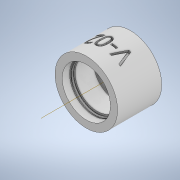
# Autodesk Inventor part: brakeStopAndOuterHousing
Saved by Autodesk Inventor 2021.1 (Build 251245000, 245)
## iProperties
Created: 2020-08-18
Part Number: brakeStopAndOuterHousing
Material: Generic
Document SubType Name: Modeling
Designer: robst
Density: 1 g/cm^3
Appearance: Default
Author: robst
Autodesk Inventor part; units mm, degrees
ref_plane "YZ Plane" through (0, 0, 0) normal (1, 0, 0) x (0, 1, 0)
ref_plane "XY Plane" through (0, 0, 0) normal (0, 0, 1) x (1, 0, 0)
sketch "Sketch3" plane through (0, 0, 0) normal (0, 0, 1) x (1, 0, 0)
  circle A0 centre (0, 0) radius 8.0645
  circle A1 centre (0, 0) radius 26.9875
  dimension "d8" = 16.129
  dimension "d9" = 53.975
  constraints: 2 centre point, 2 coincident
  measures "d8" diameter of A0
  measures "d9" diameter of A1
extrude "Extrusion3" add sketch "Sketch3" along normal blind 38.1
sketch "Sketch4" plane through (0, 0, 38.1) normal (0, 0, 1) x (1, 0, 0)
  circle A0 centre (0, 0) radius 20.7874
  dimension "d12" = 41.5747
  constraints: 1 centre point, 1 coincident
  measures "d12" diameter of A0
extrude "Extrusion4" cut sketch "Sketch4" against normal blind 25.4
sketch "Sketch5" plane through (0, 0, 0) normal (1, 0, 0) x (0, 1, 0)
  line L0 (20.7874, 38.1) -> (20.7874, 12.7) projected
  line L1 (26.9875, 38.1) -> (-26.9875, 38.1) projected
  line L2 (20.7874, 38.1) -> (20.7874, 38.1)
  line L3 (20.7874, 38.1) -> (19.6634, 37.4511)
  line L4 (19.6634, 37.2531) -> (20.7874, 36.6042)
  arc A0 (19.6634, 37.4511) -> (19.6634, 37.2531) centre (19.7206, 37.3521) ccw
  line L5 (0, -10.16) -> (0, 60.96) construction
  line L6 (20.7874, 36.6042) -> (20.7874, 38.1)
  point P0 (0, 0)
  dimension "d15" = 60
  dimension "d17" = 0.1143
  dimension "d18" = 19.6063
  dimension "d27" = 0
  constraints: 8 end point, 2 point on circle, 2 tangent, 1 centre point, 1 collinear, 1 equal length, 1 point on line, 1 vertical
  measures "d15" angle of L4 L3
  measures "d17" radius of A0
  measures "d18" distance edge to line of A0 L5
  measures "d27" distance of L2.end L0.start
coil "Coil2" sketch "Sketch5" operation add axis through (0, 0, -10) along (0, 0, -1) pitch 2.1167 turns 12 hand right
ref_plane "Work Plane1" through (0, 26.9875, 0) normal (0, 1, 0) x (-1, 0, 0)
ref_plane "Work Plane2" through (0, 26.9875, 0) normal (0, 1, 0) x (-1, 0, 0)
sketch "Sketch7" plane through (0, 26.9875, 0) normal (0, 1, 0) x (-1, 0, 0)
  line L0 (26.9875, 0) -> (26.9875, 38.1) projected
  line L1 (26.9875, 38.1) -> (-26.9875, 38.1) projected
  line L2 (-26.9875, 0) -> (-26.9875, 38.1) projected
  line L3 (-26.9875, 19.05) -> (26.9875, 19.05) construction
  line L4 (-7.4152, 25.4) -> (-11.7892, 12.7)
  line L5 (-11.7892, 12.7) -> (-13.6108, 12.7)
  line L6 (-13.6108, 12.7) -> (-17.9848, 25.4)
  line L7 (-17.9848, 25.4) -> (-16.1735, 25.4)
  line L8 (-16.1735, 25.4) -> (-12.6537, 14.851)
  line L9 (-12.6537, 14.851) -> (-9.1339, 25.4)
  line L10 (-9.1339, 25.4) -> (-7.4152, 25.4)
  line L11 (-1.765, 17.4857) -> (-6.5713, 17.4857)
  line L12 (-6.5713, 17.4857) -> (-6.5713, 19.0294)
  line L13 (-6.5713, 19.0294) -> (-1.765, 19.0294)
  line L14 (-1.765, 19.0294) -> (-1.765, 17.4857)
  spline S0 degree 2 poles (7.8269, 19.05) (7.8269, 15.6331) (5.8406, 12.4324) (3.7719, 12.4324) knots 0 0 0 1 2 2 2
  spline S1 degree 2 poles (3.7719, 12.4324) (1.6724, 12.4324) (-0.2933, 15.6949) (-0.2933, 19.0397) knots 0 0 0 1 2 2 2
  spline S2 degree 2 poles (-0.2933, 19.0397) (-0.2933, 22.4771) (1.693, 25.6573) (3.7719, 25.6573) knots 0 0 0 1 2 2 2
  spline S3 degree 2 poles (3.7719, 25.6573) (5.8611, 25.6573) (7.8269, 22.3639) (7.8269, 19.05) knots 0 0 0 1 2 2 2
  spline S4 degree 2 poles (5.645, 15.1803) (5.892, 15.8081) (6.0979, 17.7429) (6.0979, 19.05) knots 0 0 0 1 2 2 2
  spline S5 degree 2 poles (6.0979, 19.05) (6.0979, 20.3571) (5.892, 22.2816) (5.6347, 22.93) knots 0 0 0 1 2 2 2
  spline S6 degree 2 poles (5.6347, 22.93) (5.3774, 23.5784) (4.4821, 24.2473) (3.7719, 24.2473) knots 0 0 0 1 2 2 2
  spline S7 degree 2 poles (3.7719, 24.2473) (3.0618, 24.2473) (2.1458, 23.5784) (1.8782, 22.9094) knots 0 0 0 1 2 2 2
  spline S8 degree 2 poles (1.8782, 22.9094) (1.6209, 22.261) (1.4357, 20.285) (1.4357, 19.0397) knots 0 0 0 1 2 2 2
  spline S9 degree 2 poles (1.4357, 19.0397) (1.4357, 17.7018) (1.6004, 15.911) (1.868, 15.2112) knots 0 0 0 1 2 2 2
  spline S10 degree 2 poles (1.868, 15.2112) (2.115, 14.5525) (3.0309, 13.8424) (3.7719, 13.8424) knots 0 0 0 1 2 2 2
  spline S11 degree 2 poles (3.7719, 13.8424) (4.4718, 13.8424) (5.3877, 14.5113) (5.645, 15.1803) knots 0 0 0 1 2 2 2
  line L15 (17.285, 12.7) -> (9.453, 12.7)
  line L16 (9.453, 12.7) -> (9.453, 14.5011)
  spline S12 degree 2 poles (9.453, 14.5011) (10.2969, 15.2935) (11.7995, 16.7652) (12.5199, 17.5577) knots 0 0 0 1 2 2 2
  spline S13 degree 2 poles (12.5199, 17.5577) (13.971, 19.1529) (15.0311, 21.0672) (15.0311, 22.0861) knots 0 0 0 1 2 2 2
  spline S14 degree 2 poles (15.0311, 22.0861) (15.0311, 22.6212) (14.7017, 23.424) (14.4033, 23.6813) knots 0 0 0 1 2 2 2
  spline S15 degree 2 poles (14.4033, 23.6813) (14.1048, 23.9386) (13.3226, 24.1959) (12.8492, 24.1959) knots 0 0 0 1 2 2 2
  spline S16 degree 2 poles (12.8492, 24.1959) (12.3964, 24.1959) (11.4701, 23.9694) (11.0482, 23.7945) knots 0 0 0 1 2 2 2
  spline S17 degree 2 poles (11.0482, 23.7945) (10.688, 23.6504) (10.019, 23.2387) (9.8132, 23.0947) knots 0 0 0 1 2 2 2
  line L17 (9.8132, 23.0947) -> (9.7205, 23.0947)
  line L18 (9.7205, 23.0947) -> (9.7205, 24.906)
  spline S18 degree 2 poles (9.7205, 24.906) (10.2454, 25.1633) (12.1288, 25.6676) (12.9727, 25.6676) knots 0 0 0 1 2 2 2
  spline S19 degree 2 poles (12.9727, 25.6676) (14.7532, 25.6676) (16.7601, 23.7842) (16.7601, 22.1787) knots 0 0 0 1 2 2 2
  spline S20 degree 2 poles (16.7601, 22.1787) (16.7601, 21.4274) (16.4102, 20.1718) (16.1014, 19.6366) knots 0 0 0 1 2 2 2
  spline S21 degree 2 poles (16.1014, 19.6366) (15.7927, 19.0809) (14.8973, 17.99) (14.4033, 17.4651) knots 0 0 0 1 2 2 2
  spline S22 degree 2 poles (14.4033, 17.4651) (13.6005, 16.5903) (11.6348, 14.7172) (11.0482, 14.1717) knots 0 0 0 1 2 2 2
  line L19 (11.0482, 14.1717) -> (17.285, 14.1717)
  line L20 (17.285, 14.1717) -> (17.285, 12.7)
  point P0 (0, 0)
  constraints: 2 end point, 2 midpoint, 1 horizontal
emboss "Emboss1" sketch "Sketch7" operation cut depth 2.54 direction (0, -1, 0) wrap yes faces at (26.638, -4.3291, 25.4)
sketch "Sketch9" plane through (0, 0, 12.7) normal (0, 0, 1) x (1, 0, 0)
  circle A0 centre (0, 0) radius 20.7874
  circle A1 centre (0, 0) radius 19.177
  dimension "d51" = 41.5747
  dimension "d52" = 38.354
  constraints: 2 centre point, 2 coincident
  measures "d51" diameter of A0
  measures "d52" diameter of A1
extrude "Extrusion5" add sketch "Sketch9" along normal blind 15.875
sketch "Sketch10" plane through (0, 0, 38.1) normal (0, 0, 1) x (1, 0, 0)
  circle A0 centre (0, 0) radius 20.7874
  dimension "d55" = 41.5747
  constraints: 1 centre point, 1 coincident
  measures "d55" diameter of A0
extrude "Extrusion6" cut sketch "Sketch10" against normal blind 6.35
equation "\"d8\" = innerDiameter"
equation "\"d9\" = outsideDiameter"
equation "\"d10\" = lengthOfBrakeStop"
equation "\"d12\" = b1MajorDiameterAvg"
equation "\"d13\" = depthOfThread"
equation "\"d17\" = b1RootRadiusAvg"
equation "\"d18\" = 0.5 * b1MinorDiameterAvg"
equation "\"d28\" = pitch"
equation "\"d29\" = depthOfThread"
equation "\"d51\" = b1MajorDiameterAvg"
equation "\"d55\" = b1MajorDiameterAvg"
equation "\"innerDiameter\" = 16.129"
equation "\"heightOfBrake\" = 6.35"
equation "\"majorDiameter\" = 41.22928"
equation "\"pitchDiameter\" = 39.85514"
equation "\"minorDiameter\" = 38.7096"
equation "\"crestFlat\" = 0.4318"
equation "\"rootRadius\" = 0.22352"
equation "\"threadDepth\" = 1.52146"
equation "\"outsideDiameter\" = 53.975"
equation "\"lengthOfBrakeStop\" = 38.1"
equation "\"depthOfThread\" = lengthOfBrakeStop - brakeStopLength"
equation "\"d36\" = 0.5 * outsideDiameter"
equation "\"brakeStopLength\" = 12.7"
equation "\"d48\" = 0.5 * outsideDiameter"
equation "\"b1MajorDiameterAvg\" = 41.57472"
equation "\"b1MinorDiameterAvg\" = 39.21252"
equation "\"b1RootRadiusAvg\" = 0.1143"
equation "\"pitch\" = 2.116667"
body "Solid2"
